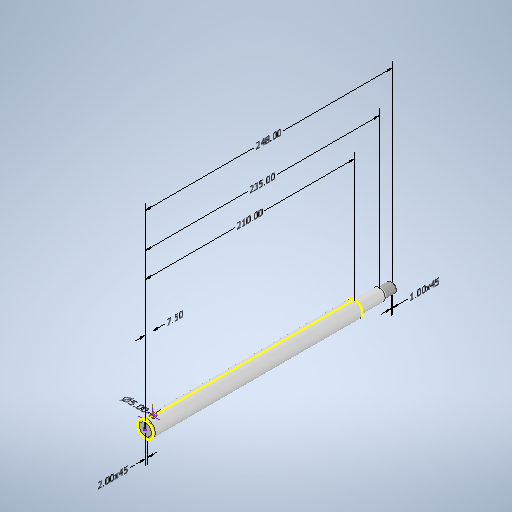
# Autodesk Inventor part: Część1
Saved by Autodesk Inventor 2025.2 (Build 292293000, 293)
## iProperties
Created: 2025-03-17
Part Number: Część1
Material: Ogólny
Document SubType Name: Modeling
Designer: marci
Density: 1 g/cm^3
Appearance: Domyślna
Author: marci
Autodesk Inventor part; units mm, degrees
ref_plane "YZ Plane" through (0, 0, 0) normal (1, 0, 0) x (0, 1, 0)
ref_plane "XZ Plane" through (0, 0, 0) normal (0, 1, 0) x (-1, 0, 0)
ref_plane "XY Plane" through (0, 0, 0) normal (0, 0, 1) x (1, 0, 0)
sketch "Szkic1" plane through (0, 0, 0) normal (0, 0, 1) x (1, 0, 0)
  circle A0 centre (0, 0) radius 8
  dimension "d0" = 16
  constraints: 1 centre point, 1 coincident
  measures "d0" diameter of A0
extrude "Wyciągnięcie proste1" add sketch "Szkic1" against normal blind 210
sketch "Szkic2" plane through (0, 0, 0) normal (0, 0, 1) x (1, 0, 0)
  line L0 (0, 0) -> (0, 8)
  circle A0 centre (0, 0) radius 8 projected
  circle A1 centre (0, 0) radius 8 projected
  circle A2 centre (0, 0) radius 8 projected
  constraints: 2 end point, 1 vertical, 1 vertical alignment, 1 other
sketch3d "Szkic 3D1"
sketch "Szkic3" plane through (0, 0, 0) normal (0, 0, 1) x (1, 0, 0)
  circle A0 centre (0, 0) radius 8
  circle A1 centre (0, 0) radius 8
  point P0 (0, 8)
  constraints: 3 centre point
sketch3d "Szkic 3D2"
sketch "Szkic4" plane through (0, 0, 0) normal (0, 0, 1) x (1, 0, 0)
  circle A0 centre (0, 0) radius 8 projected
  circle A1 centre (0, 0) radius 8 projected
  point P0 (0, 8)
hole "Otwór1" at (0, 8, -7.5) direction (0, -1, 0) diameter 5 end through all
chamfer "Faza2" distance 2 angle 45 1 edges at (-8, 0, 0)
sketch "Szkic6" plane through (0, 0, -210) normal (0, 0, -1) x (-1, 0, 0)
  point P0 (0, 0)
sketch "Szkic7" plane through (0, 0, -210) normal (0, 0, -1) x (-1, 0, 0)
  circle A0 centre (0, 0) radius 6
  constraints: 1 centre point, 1 coincident
extrude "Wyciągnięcie proste2" add sketch "Szkic7" along normal blind 25
sketch "Szkic8" plane through (0, 0, -235) normal (0, 0, -1) x (-1, 0, 0)
  circle A0 centre (0, 0) radius 5
  constraints: 1 centre point, 1 coincident
extrude "Wyciągnięcie proste3" add sketch "Szkic8" along normal blind 13
chamfer "Faza3" distance 1 angle 45 1 edges at (5, 0, -248)
thread "Gwint1" size "M10x1.5" class "6g" standard "ANSI Metric M Profile" length 10
